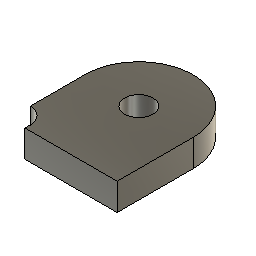
Support Arm Attachment left Final v6 (Autodesk Fusion 360 archive; units mm, degrees)
design "Arm travel stop left"
Autodesk Fusion 360 part; units mm, degrees
sketch "Sketch1" plane through (0, 0, 0) normal (0, 0, 1) x (1, 0, 0)
  line L0 (0, 0) -> (0, 14)
  line L1 (0, 0) -> (20, 0)
  line L2 (10, 0) -> (10, 14) construction
  line L3 (20, 0) -> (20, 14)
  arc A0 (20, 14) -> (0, 14) centre (10, 14) ccw
  circle A1 centre (10, 14) radius 2.6
  dimension "d1" = 14
  dimension "d2" = 20
  dimension "d3" = 14
  dimension "d4" = 14
  dimension "d5" = 5.2
  constraint coincident L0.start L1.start
  constraint vertical L0
  constraint horizontal L1
  constraint midpoint L1 L2.start
  constraint perpendicular L1 L2
  constraint perpendicular L1 L3
  constraint coincident L2.end A0.centre
  measures "d1" distance of L0.start L0.end
  measures "d2" distance of L0.start L1.end
  measures "d3" distance of L2.start L2.end
  measures "d4" distance of L1.end L3.end
  measures "d5" diameter of A1
extrude "Extrude1" add sketch "Sketch1" along normal blind 5
sketch "Sketch2" plane through (0, 0, 5) normal (0, 0, 1) x (-1, 0, 0)
  circle A0 centre (-10, -14) radius 2.6
  line L0 (0, 0) -> (-20, 0)
  line L1 (-20, 0) -> (-20, -14)
  arc A1 (-20, -14) -> (0, -14) centre (-10, -14) ccw
  line L2 (0, -14) -> (0, 0)
  circle A2 centre (-10, -14) radius 6 construction
  line L3 (-10, -14) -> (-5.7574, -9.7574) construction
  line L4 (-10, -14) -> (-4, -14) construction
  line L5 (-10, -14) -> (-14.2426, -9.7574) construction
  line L6 (-10, -14) -> (-14.2426, -18.2426) construction
  line L7 (-10, -14) -> (-5.7574, -18.2426) construction
  dimension "d8" = 12
  dimension "d9" = 45
  constraint concentric A0 A2
  constraint horizontal L4
  constraint coincident A0.centre A1.centre
  constraint coincident A2 L3.end
  constraint coincident A2 L5.end
  constraint perpendicular L3 L5
  constraint coincident A2 L6.end
  constraint perpendicular L5 L6
  constraint coincident A2 L7.end
  constraint perpendicular L6 L7
  measures "d8" diameter of A2
  measures "d9" angle of L3 L4
hole "Hole1" [suppressed]
sketch "Sketch3" plane through (0, 0, 0) normal (0, 0, -1) x (1, 0, 0)
  circle A0 centre (10, -14) radius 2.6
  line L0 (20, 0) -> (0, 0)
  line L1 (0, 0) -> (0, -14)
  arc A1 (0, -14) -> (20, -14) centre (10, -14) ccw
  line L2 (20, -14) -> (20, 0)
  circle A2 centre (10, -14) radius 10 construction
  line L3 (10, -24) -> (10, -4) construction
  point P0 (10, -7.875)
  dimension "d33" = 20
  dimension "d51" = 6.125
  constraint concentric A0 A2
  constraint midpoint A1 L3.start
  constraint coincident A2 L3.end
  constraint vertical L3
  constraint coincident L3 P0
  measures "d33" diameter of A2
  measures "d51" distance of A0.centre P0
hole "Hole5" [suppressed]
thread "Thread2" [suppressed]
sketch "Sketch7" plane through (0, 0, 0) normal (0, 0, -1) x (1, 0, 0)
  circle A0 centre (10, -14) radius 2.6
  line L0 (20, 0) -> (0, 0)
  line L1 (0, 0) -> (0, -14)
  arc A1 (0, -14) -> (20, -14) centre (10, -14) ccw
  line L2 (20, -14) -> (20, 0)
  line L3 (0, 0) -> (0, -4) construction
  line L4 (0, 0) -> (3, 0) construction
  line L5 (3, 0) -> (3, -1)
  arc A2 (0, -4) -> (3, -1) centre (0, -1) ccw
  dimension "d44" = 4
  dimension "d45" = 3
  dimension "d49" = 1
  dimension "d50" = 3
  constraint coincident L0.end L1.start
  constraint perpendicular L0 L3
  constraint perpendicular L3 L4
  constraint perpendicular L0 L5
  constraint tangent L5 A2
  measures "d44" distance of L0.end L3.end
  measures "d45" distance of L0.end L4.end
  measures "d49" distance of L4.end L5.end
  measures "d50" radius of A2
extrude "Extrude2" cut sketch "Sketch7" against normal blind 5 contours L0 L1 L5 A2
